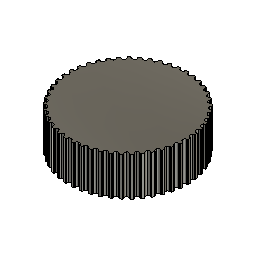
gear_49z (Autodesk Fusion 360 design; units mm, degrees)
Autodesk Fusion 360 part; units mm, degrees
sketch "Sketch1" plane through (0, 0, 0) normal (0, 0, 1) x (1, 0, 0) in component "gt2 pulley"
  circle A0 centre (0, 0) radius 15.5972 construction
  circle A1 centre (0, 0) radius 14.5932 construction
  line L0 (0, 0) -> (0, 15.5972) construction
  line L1 (0, 0) -> (0.9993, 15.5651) construction
  line L2 (0, 0) -> (1.4073, 15.5336) construction
  circle A2 centre (0, 0) radius 15.3432 construction
  arc A3 (0.3874, 15.203) -> (0.4544, 14.9131) centre (1.3844, 15.2806) ccw
  circle A4 centre (0, 0) radius 15.1932 construction
  arc A5 (0.2402, 15.3413) -> (0, 15.3432) centre (0, 0) ccw
  arc A6 (0.3874, 15.203) -> (0.2402, 15.3413) centre (0.2379, 15.1913) ccw
  arc A7 (0.4544, 14.9131) -> (0.935, 14.5632) centre (0.9705, 15.1171) ccw
  arc A8 (0, 15.3432) -> (-0.2402, 15.3413) centre (0, 0) ccw
  arc A9 (-0.2402, 15.3413) -> (-0.3874, 15.203) centre (-0.2379, 15.1913) ccw
  arc A10 (-0.4544, 14.9131) -> (-0.3874, 15.203) centre (-1.3844, 15.2806) ccw
  arc A11 (-0.935, 14.5632) -> (-0.4544, 14.9131) centre (-0.9705, 15.1171) ccw
  arc A12 (0.935, 14.5632) -> (-0.935, 14.5632) centre (0, 0) ccw
  point P0 (1.3844, 15.2806)
  point P1 (0, 15.3432)
  dimension "d18" = 31.831
  dimension "d19" = 3.6
  dimension "d22" = 1.004
  dimension "d24" = 0.75
  dimension "d26" = 1
  dimension "d27" = 0.15
  dimension "d28" = 0.15
  dimension "d47" = 0.555
  dimension "d52" = 3.812
  constraint coincident A0.centre A1.centre
  constraint coincident A0 L0.end
  constraint vertical L0
  constraint coincident A0 L1.end
  constraint coincident A0 L2.end
  constraint concentric A1 A2
  constraint coincident A1 A7.end
  constraint coincident L1 A7.end
  constraint coincident A2 P0
  constraint coincident L2 P0
  constraint coincident P0 A3.centre
  constraint coincident A2 P1
  constraint coincident L0 P1
  constraint concentric A2 A4
  constraint coincident P1 A5.end
  constraint coincident A4 A6.centre
  constraint coincident A3.start A6.start
  constraint tangent A3 A6
  constraint tangent A3 A7
  constraint symmetric L0 A7.end A11.start
  constraint symmetric L0 A3.start A9.end
  constraint symmetric L0 A3.end A10.start
  constraint symmetric L0 A3 A10
  constraint symmetric L0 A5.start A8.end
  constraint symmetric L0 P1 A5.end
  constraint symmetric L0 A5 A8
  constraint symmetric L0 A6 A9
  constraint symmetric L0 A7 A11
  constraint coincident A1 A11.start
  constraint tangent A1 A7
  constraint coincident L1 A7.centre
  measures "d22" distance of A0 A1
  measures "d24" distance of A1 A2
  measures "d26" radius of A3
  measures "d27" distance of A2 A4
  measures "d28" radius of A6
  measures "d47" radius of A7
extrude "Extrude1" add sketch "Sketch1" along normal blind 10 makes body 1
pattern_circular "C-Pattern1" count 49 over 360 about axis through (0, 0, 1.75) along (0, 0, 1) of bodies 1 makes body 2 at (-1.9692, 14.4597, 6.6667) makes body 3 at (-4.4007, 13.9139, 6.6667) makes body 4 at (-6.1438, 13.2369, 6.6667) makes body 5 at (-7.786, 12.3425, 6.6667) makes body 6 at (-8.1345, 12.1157, 3.3333) makes body 7 at (-10.2267, 10.4104, 6.6667) makes body 8 at (-11.8488, 8.5187, 6.6667) makes body 9 at (-12.5328, 7.4759, 6.6667) makes body 10 at (-13.6221, 5.2346, 6.6667) makes body 11 at (-14.1796, 3.4496, 6.6667) makes body 12 at (-14.4224, 2.2264, 6.6667) makes body 13 at (-14.5442, 1.1942, 3.3333) makes body 14 at (-14.5154, -1.5047, 6.6667) makes body 15 at (-14.0477, -3.9524, 6.6667) makes body 16 at (-13.427, -5.7164, 6.6667) makes body 17 at (-12.8899, -6.8419, 6.6667) makes body 18 at (-11.5379, -8.9352, 6.6667) makes body 19 at (-10.3005, -10.3373, 6.6667) makes body 20 at (-9.3803, -11.179, 6.6667) makes body 21 at (-7.8738, -12.2868, 6.6667) makes body 22 at (-5.6685, -13.4473, 6.6667) makes body 23 at (-3.9023, -14.0617, 6.6667) makes body 24 at (-3.5001, -14.1672, 3.3333) makes body 25 at (-1.6597, -14.4985, 3.3333) makes body 26 at (0.2079, -14.5917, 3.3333) makes body 27 at (2.8916, -14.3038, 6.6667) makes body 28 at (5.2831, -13.6033, 6.6667) makes body 29 at (6.9793, -12.816, 6.6667) makes body 30 at (8.048, -12.1733, 6.6667) makes body 31 at (9.5386, -11.0442, 6.6667) makes body 32 at (10.3005, -10.3373, 3.3333) makes body 33 at (12.3702, -7.742, 6.6667) makes body 34 at (12.9861, -6.6576, 6.6667) makes body 35 at (13.427, -5.7164, 6.6667) makes body 36 at (14.2038, -3.3486, 6.6667) makes body 37 at (14.5775, -0.6755, 6.6667) makes body 38 at (14.582, 0.5716, 6.6667) makes body 39 at (14.5043, 1.6081, 6.6667) makes body 40 at (13.9601, 4.2517, 6.6667) makes body 41 at (13.0332, 6.5649, 6.6667) makes body 42 at (12.8408, 6.9336, 3.3333) makes body 43 at (11.4739, 9.0172, 6.6667) makes body 44 at (9.6171, 10.976, 6.6667) makes body 45 at (8.1345, 12.1157, 6.6667) makes body 46 at (7.786, 12.3426, 3.3333) makes body 47 at (4.7953, 13.7828, 6.6667) makes body 48 at (4.4006, 13.9139, 3.3333) makes body 49 at (2.5853, 14.3624, 3.3333)
sketch "Sketch2" plane through (0, 0, 10) normal (0, 0, 1) x (-1, 0, 0)
  arc A0 (-15.0699, -2.0439) -> (-15.183, -2.2114) centre (-15.0346, -2.1897) ccw
  arc A1 (-15.183, -2.2114) -> (-15.1063, -2.6856) centre (0, 0) ccw
  arc A2 (-15.1063, -2.6856) -> (-14.9463, -2.8089) centre (-14.9586, -2.6594) ccw
  arc A3 (-14.6494, -2.8287) -> (-14.9463, -2.8089) centre (-14.8638, -3.8054) ccw
  arc A4 (-14.2273, -3.2473) -> (-14.6494, -2.8287) centre (-14.7684, -3.3708) ccw
  arc A5 (-14.5258, -1.4013) -> (-14.2273, -3.2473) centre (0, 0) ccw
  arc A6 (-14.7945, -1.9316) -> (-14.5258, -1.4013) centre (-15.0782, -1.4546) ccw
  arc A7 (-15.0699, -2.0439) -> (-14.7945, -1.9316) centre (-15.3057, -1.0721) ccw
  circle A8 centre (0, 0) radius 14.5932
  constraint concentric A1 A8
extrude "Extrude2" add sketch "Sketch2" against normal blind 10 contours A5 A8 bodies 1 2 3 4 5 6 7 8 9 10 11 12 13 14 15 16 17 18 19 20 21 22 23 24 25 26 27 28 29 30 31 32 33 34 35 36 37 38 39 40 41 42 43 44 45 46 47 48 49
extrude "Extrude4" [suppressed] in component "gt2 pulley"
pattern_circular "C-Pattern7" [suppressed] in component "gt2 pulley"
extrude "Extrude3" [suppressed] in component "gt2 pulley"
pattern_circular "C-Pattern6" [suppressed] in component "gt2 pulley"
extrude "Extrude2'" [suppressed] in component "gt2 pulley"
pattern_circular "C-Pattern5" [suppressed] in component "gt2 pulley"
extrude "Extrude1'" [suppressed] in component "gt2 pulley"
pattern_circular "C-Pattern4" [suppressed] in component "gt2 pulley"
pattern_circular "C-Pattern3" [suppressed] in component "gt2 pulley"
pattern_circular "C-Pattern2" [suppressed] in component "gt2 pulley"
pattern_circular "C-Pattern1'" [suppressed] in component "gt2 pulley"
copy_body "Body->Comp1" [suppressed] in component "Component"
copy_body "Body->Comp2" [suppressed] in component "Component'"
copy_body "Body->Comp3" [suppressed] in component "Component''"
copy_body "Body->Comp4" [suppressed] in component "Component'''"
copy_body "Body->Comp5" [suppressed] in component "Component''''"
copy_body "Body->Comp6" [suppressed] in component "Component'''''"
copy_body "Body->Comp7" [suppressed] in component "Component''''''"
copy_body "Body->Comp8" [suppressed] in component "Component'''''''"
copy_body "Body->Comp9" [suppressed] in component "Component''''''''"
copy_body "Body->Comp10" [suppressed] in component "Component'''''''''"
copy_body "Body->Comp11" [suppressed] in component "Component''''''''''"
copy_body "Body->Comp12" [suppressed] in component "Component'''''''''''"
copy_body "Body->Comp13" [suppressed] in component "Component''''''''''''"
copy_body "Body->Comp14" [suppressed] in component "Component'''''''''''''"
copy_body "Body->Comp15" [suppressed] in component "Component''''''''''''''"
copy_body "Body->Comp16" [suppressed] in component "Component'''''''''''''''"
copy_body "Body->Comp17" [suppressed] in component "Component''''''''''''''''"
copy_body "Body->Comp18" [suppressed] in component "Component'''''''''''''''''"
copy_body "Body->Comp19" [suppressed] in component "Component''''''''''''''''''"
copy_body "Body->Comp20" [suppressed] in component "Component'''''''''''''''''''"
component "gt2 pulley" placed x (1, 0, 0) y (0, 1, 0) z (0, 0, 1) at (0, 0, 0)
equation "NumTeeth = 50" comment "min 20"
equation "ToothPitch = 2 mm"
equation "PullyDia = NumTeeth * ToothPitch / PI"
equation "ToothAng = ( ( 360 / NumTeeth ) * 1 deg )"
equation "TransOffsetAngle = ToothAng * 0.2"
equation "Sholulder_Radius = 0.15 mm"
equation "Root_Radius = 0.555 mm"
equation "TransRadius = 1 mm"
equation "ToolHeight = 0.75 mm"
equation "PLD = 0.254 mm"
equation "d18 = PullyDia"
equation "d19 = ToothAng / 2"
equation "d22 = PLD + ToolHeight"
equation "d24 = ToolHeight"
equation "d26 = TransRadius"
equation "d27 = Sholulder_Radius"
equation "d31 = NumTeeth"
equation "d33 = NumTeeth"
equation "d35 = NumTeeth"
equation "d37 = NumTeeth"
equation "d41 = NumTeeth"
equation "d45 = NumTeeth"
equation "d47 = Root_Radius"
equation "d50 = NumTeeth"
